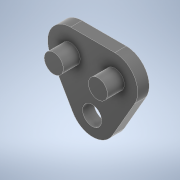
# Autodesk Inventor part: Pieza5
Saved by Autodesk Inventor 2022 (Build 260153000, 153)
## iProperties
Created: 2022-11-04
Part Number: Pieza5
Material: Resina acetálica, negra
Document SubType Name: Modeling
Designer: Mauricio Guerrero
Density: 1.425 g/cm^3
Appearance: Suave - Negro
Author: Mauricio Guerrero
## iProperties of the stored document Pieza5_3DPrint.ipt
Created: 2022-11-06
Part Number: Pieza5_3DPrint
Material: Genérico
Document SubType Name: Modeling
Designer: Mauricio Guerrero
Density: 1 g/cm^3
Appearance: Valor por defecto
Author: Mauricio Guerrero
Autodesk Inventor part; units mm, degrees
ref_plane "YZ Plane" through (0, 0, 0) normal (1, 0, 0) x (0, 1, 0)
ref_plane "XZ Plane" through (0, 0, 0) normal (0, 1, 0) x (-1, 0, 0)
ref_plane "XY Plane" through (0, 0, 0) normal (0, 0, 1) x (1, 0, 0)
sketch "Boceto1" plane through (0, 0, 0) normal (0, 0, 1) x (1, 0, 0)
  circle A0 centre (6.9411, 0.443) radius 1.25
  circle A1 centre (13.2811, 0.443) radius 1.25
  line L0 (6.9411, 0.443) -> (13.2811, 0.443) construction
  circle A2 centre (10.1111, -5.037) radius 1.25
  line L1 (7.2902, 3.563) -> (13.0745, 3.563)
  line L2 (4.6921, -0.937) -> (7.5843, -5.9464)
  line L3 (12.7804, -5.9464) -> (15.6726, -0.937)
  arc A3 (7.2902, 3.563) -> (4.6921, -0.937) centre (7.2902, 0.563) ccw
  arc A4 (15.6726, -0.937) -> (13.0745, 3.563) centre (13.0745, 0.563) ccw
  arc A5 (7.5843, -5.9464) -> (12.7804, -5.9464) centre (10.1824, -4.4464) ccw
  dimension "d2" = 2.5
  dimension "d9" = 2.5
  dimension "d10" = 6.34
  dimension "d13" = 2.5
  dimension "d14" = 5.48
  dimension "d15" = 3.12
  dimension "d16" = 60
  dimension "d17" = 60
  dimension "d18" = 60
  dimension "d19" = 3
  constraints: 8 end point, 6 centre point, 6 point on circle, 6 tangent, 2 equal radius, 2 horizontal, 1 horizontal alignment
  measures "d2" diameter of A0
  measures "d9" diameter of A1
  measures "d10" distance of L0.end L0.start
  measures "d13" diameter of A2
  measures "d14" distance from line of A2.centre L0
  measures "d15" distance between parallel lines of L1 L0
  measures "d16" angle of L1 L2
  measures "d17" angle of L3 L1
  measures "d18" angle of L3 L2
  measures "d19" radius of A3
extrude "Extrusión1" add sketch "Boceto1" along normal blind 1.5 contours A0 | A1 | L1 A4 L3 A5 L2 A3
sketch "Boceto3" plane through (0, 0, 1.5) normal (0, 0, 1) x (1, 0, 0)
  arc A0 (7.2902, 3.563) -> (4.6921, -0.937) centre (7.2902, 0.563) ccw projected
  circle A1 centre (7.2902, 0.563) radius 1.25
  arc A2 (15.6726, -0.937) -> (13.0745, 3.563) centre (13.0745, 0.563) ccw projected
  circle A3 centre (13.0745, 0.563) radius 1.25
  point P0 (0, 0)
  dimension "d22" = 2.5
  dimension "d23" = 2.5
  constraints: 2 centre point, 2 coincident
  measures "d22" diameter of A1
  measures "d23" diameter of A3
extrude "Extrusión2" add sketch "Boceto3" along normal blind 2.2
